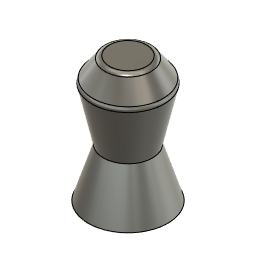
forme4proto v2 (Autodesk Fusion 360 design; units mm, degrees)
Autodesk Fusion 360 part; units mm, degrees
sketch "Esquisse1" plane through (0, 0, 0) normal (0, 0, 1) x (1, 0, 0)
  line L0 (0, 0) -> (-65, 0)
  line L1 (-65, 0) -> (-40, 80)
  line L2 (-40, 80) -> (-60, 170)
  line L3 (-60, 170) -> (-35, 205)
  line L4 (-35, 205) -> (0, 205)
  line L5 (0, 205) -> (0, 0)
  dimension "d1" = 65
  dimension "d3" = 35
  dimension "d4" = 90
  dimension "d5" = 80
  dimension "d6" = 40
  dimension "d7" = 60
  dimension "d8" = 35
  constraint coincident L0.start L5.end
  constraint horizontal L0
  constraint horizontal L4
  constraint perpendicular L0 L5
  measures "d1" distance of L0.start L0.end
  measures "d3" vertical distance of L2.end L3.end
  measures "d4" vertical distance of L1.end L2.end
  measures "d5" vertical distance of L0.end L1.end
  measures "d6" distance of L1.end L5
  measures "d7" distance of L2.end L5
  measures "d8" distance of L3.end L4.end
revolve "Révolution1" add sketch "Esquisse1" angle 360 about axis through (0, 205, 0) along (0, -1, 0)
fillet "Congé1" radius 9 1 edges at (-55.9396, 170, 21.6969)
fillet "Congé2" radius 9 1 edges at (-32.6315, 205, 12.6565)
shell "Coque1" thickness 2 removed faces 1 at (20.2416, 0, -0.2148)
